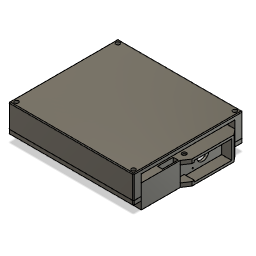
gboard_cap (Autodesk Fusion 360 design; units mm, degrees)
Autodesk Fusion 360 part; units mm, degrees
sketch "草图1" plane through (0, 0, 0) normal (0, 1, 0) x (1, 0, 0)
  line L0 (0, 0) -> (0, -50) construction
  line L1 (0, -50) -> (70, -50)
  line L2 (80, -60) -> (-80, -60)
  line L3 (-70, -50) -> (0, -50)
  line L4 (-70, 50) -> (70, 50)
  line L5 (80, 60) -> (-80, 60)
  line L6 (-70, 50) -> (-70, -50)
  line L7 (70, 50) -> (70, -50)
  line L8 (-80, 60) -> (-80, -60)
  line L9 (80, 60) -> (80, -60)
  line L10 (0, 0) -> (70, 0) construction
  line L11 (-70, 60) -> (-70, 65)
  line L12 (-70, 65) -> (-60, 65)
  line L13 (-60, 65) -> (-60, 60)
  line L14 (70, 60) -> (70, 65)
  line L15 (70, 65) -> (60, 65)
  line L16 (60, 65) -> (60, 60)
  line L17 (-70, -60) -> (-70, -65)
  line L18 (-70, -65) -> (-60, -65)
  line L19 (-60, -65) -> (-60, -60)
  line L20 (70, -60) -> (70, -65)
  line L21 (70, -65) -> (60, -65)
  line L22 (60, -65) -> (60, -60)
  dimension "d5" = 50
  dimension "d21" = 160
  dimension "d23" = 140
  dimension "d24" = 100
  dimension "d25" = 10
  dimension "d26" = 120
  dimension "d27" = 10
  dimension "d28" = 70
  dimension "d31" = 5
  dimension "d32" = 10
  dimension "d33" = 10
  dimension "d34" = 10
  dimension "d35" = 10
  dimension "d36" = 5
  dimension "d37" = 5
  dimension "d38" = 10
  dimension "d39" = 10
  dimension "d40" = 5
  dimension "d41" = 10
  dimension "d42" = 10
  constraint coincident L0.start L10.start
  constraint vertical L0
  constraint perpendicular L0 L1
  constraint perpendicular L0 L3
  constraint perpendicular L3 L6
  constraint perpendicular L1 L7
  constraint perpendicular L2 L8
  constraint perpendicular L5 L9
  constraint midpoint L7 L10.end
  constraint coincident L5 L11.start
  constraint perpendicular L5 L11
  constraint perpendicular L11 L12
  constraint coincident L5 L13.end
  constraint perpendicular L5 L13
  constraint coincident L5 L14.start
  constraint perpendicular L5 L14
  constraint perpendicular L14 L15
  constraint coincident L5 L16.end
  constraint perpendicular L5 L16
  constraint coincident L2 L17.start
  constraint perpendicular L2 L17
  constraint perpendicular L17 L18
  constraint coincident L2 L19.end
  constraint perpendicular L2 L19
  constraint coincident L2 L20.start
  constraint perpendicular L2 L20
  constraint perpendicular L20 L21
  constraint coincident L2 L22.end
  constraint perpendicular L2 L22
  measures "d5" distance of L0.start L0.end
  measures "d21" distance of L5.start L5.end
  measures "d23" distance of L6 L7
  measures "d24" distance of L3 L4
  measures "d25" distance of L7 L9
  measures "d26" distance of L2 L5
  measures "d27" distance of L4 L5
  measures "d28" distance of L0.start L10.end
  measures "d31" distance of L11.start L11.end
  measures "d32" distance of L11.end L12.end
  measures "d33" distance of L8 L11
  measures "d34" distance of L14 L16
  measures "d35" distance of L9 L14
  measures "d36" distance of L5 L15
  measures "d37" distance of L2 L21
  measures "d38" distance of L20 L22
  measures "d39" distance of L9 L20
  measures "d40" distance of L18.end L19.end
  measures "d41" distance of L17 L19
  measures "d42" distance of L8 L17
extrude "拉伸4" add sketch "草图1" along normal blind 30 makes body 1
sketch "草图6" plane through (80, 0, 0) normal (1, 0, 0) x (0, 0, -1)
  line L0 (-60, 0) -> (60, 0)
  line L1 (60, 0) -> (60, 30)
  line L2 (60, 30) -> (-60, 30)
  line L3 (-60, 30) -> (-60, 0)
  line L4 (50, 3) -> (2, 3)
  line L5 (2, 3) -> (2, 27)
  line L6 (2, 27) -> (50, 27)
  line L7 (50, 27) -> (50, 3)
  line L8 (53, 30) -> (53, 0)
  line L9 (53, 0) -> (-1, 0)
  line L10 (-1, 0) -> (-1, 30)
  line L11 (-1, 30) -> (53, 30)
  dimension "d65" = 48
  dimension "d66" = 24
  dimension "d67" = 10
  dimension "d68" = 3
  dimension "d71" = -3
  constraint horizontal L4
  constraint vertical L5
  constraint horizontal L6
  constraint vertical L7
  measures "d65" distance of L4.start L4.end
  measures "d66" distance of L4.start L6.end
  measures "d67" distance of L1 L7
  measures "d68" distance of L2 L6
extrude "拉伸9" cut sketch "草图6" against normal blind 7 contours L4 L5 L6 L7 bodies 1
extrude "拉伸10" add sketch "草图6" along normal blind 6 contours L0 L2 L8 L9 L10 L11 bodies 1
sketch "草图7" plane through (73, 0, 0) normal (1, 0, 0) x (0, 0, -1)
  line L0 (50, 27) -> (2, 27)
  line L1 (2, 27) -> (2, 3)
  line L2 (2, 3) -> (50, 3)
  line L3 (50, 3) -> (50, 27)
  line L4 (2, 15) -> (50, 15) construction
  circle A0 centre (26, 15) radius 7.5
  line L5 (50, 15) -> (13, 15) construction
  line L6 (13, 15) -> (13, 27) construction
  circle A1 centre (13, 23.5) radius 0.75
  circle A2 centre (13, 6.5) radius 0.75
  line L7 (13, 15) -> (13, 6.5) construction
  dimension "d74" = 15
  dimension "d81" = 37
  dimension "d82" = 1.5
  dimension "d83" = 3.5
  dimension "d84" = 1.5
  dimension "d85" = 3.5
  constraint midpoint L1 L4.start
  constraint midpoint L3 L4.end
  constraint midpoint L4 A0.centre
  constraint perpendicular L3 L5
  constraint coincident L0 L6.end
  constraint perpendicular L0 L6
  constraint coincident L6 A1.centre
  constraint coincident A2.centre L7.end
  constraint perpendicular L4 L7
  measures "d74" diameter of A0
  measures "d81" distance of L4.end L5.end
  measures "d82" diameter of A1
  measures "d83" distance of L0 A1.centre
  measures "d84" diameter of A2
  measures "d85" distance of L2 A2.centre
extrude "拉伸11" cut sketch "草图7" against normal blind 3 contours A0 | A1 | A2 bodies 1
sketch "草图8" plane through (0, 0, 1) normal (0, 0, 1) x (1, 0, 0)
  line L0 (80, 30) -> (80, 0)
  line L1 (80, 0) -> (86, 0)
  line L2 (86, 0) -> (86, 30)
  line L3 (86, 30) -> (80, 30)
  line L4 (86, 25) -> (80, 25)
  line L5 (80, 25) -> (80, 5)
  line L6 (80, 5) -> (86, 5)
  line L7 (86, 5) -> (86, 25)
  dimension "d77" = 5
  dimension "d78" = 5
  constraint horizontal L4
  constraint vertical L5
  constraint horizontal L6
  constraint vertical L7
  constraint coincident L0 L5.end
  constraint coincident L2 L4.start
  measures "d77" distance of L3 L4
  measures "d78" distance of L1 L6
extrude "拉伸12" cut sketch "草图8" against normal blind 3 contours L0 L2 L4 L5 L6 L7 bodies 1
sketch "草图9" plane through (0, 30, 0) normal (0, 1, 0) x (-1, 0, 0)
  line L0 (70, 50) -> (70, -50)
  line L1 (70, -50) -> (-70, -50)
  line L2 (-70, -50) -> (-70, 50)
  line L3 (-70, 50) -> (70, 50)
  line L4 (-80, -60) -> (-70, -60)
  line L5 (-70, -60) -> (-70, -65)
  line L6 (-70, -65) -> (-60, -65)
  line L7 (-60, -65) -> (-60, -60)
  line L8 (-60, -60) -> (60, -60)
  line L9 (60, -60) -> (60, -65)
  line L10 (60, -65) -> (70, -65)
  line L11 (70, -65) -> (70, -60)
  line L12 (70, -60) -> (80, -60)
  line L13 (80, -60) -> (80, 60)
  line L14 (80, 60) -> (70, 60)
  line L15 (70, 60) -> (70, 65)
  line L16 (70, 65) -> (60, 65)
  line L17 (60, 65) -> (60, 60)
  line L18 (60, 60) -> (-60, 60)
  line L19 (-60, 60) -> (-60, 65)
  line L20 (-60, 65) -> (-70, 65)
  line L21 (-70, 65) -> (-70, 60)
  line L22 (-70, 60) -> (-80, 60)
  line L23 (-80, 60) -> (-80, 1)
  line L24 (-80, 1) -> (-86, 1)
  line L25 (-86, 1) -> (-86, -53)
  line L26 (-86, -53) -> (-80, -53)
  line L27 (-80, -53) -> (-80, -60)
  line L28 (-72, 11) -> (-78.2, 11)
  line L29 (-78.2, 11) -> (-78.2, 31)
  line L30 (-78.2, 31) -> (-72, 31)
  line L31 (-72, 31) -> (-72, 11)
  line L32 (-77.2, 12) -> (-77.2, 30)
  line L33 (-77.2, 30) -> (-73, 30)
  line L34 (-73, 30) -> (-73, 12)
  line L35 (-73, 12) -> (-77.2, 12)
  dimension "d86" = 6.2
  dimension "d87" = 20
  dimension "d88" = 11
  dimension "d89" = 2
  dimension "d92" = 1
  constraint horizontal L28
  constraint vertical L29
  constraint horizontal L30
  constraint vertical L31
  measures "d86" distance of L28.start L28.end
  measures "d87" distance of L28.start L30.end
  measures "d88" distance of origin L28
  measures "d89" distance of L2 L31
extrude "拉伸13" cut sketch "草图9" against normal blind 10 contours L28 L29 L30 L31 | L32 L33 L34 L35 bodies 1
extrude "拉伸14" cut sketch "草图9" against normal blind 25 contours L32 L33 L34 L35 bodies 1
sketch "草图10" plane through (0, 0, -2) normal (0, 0, -1) x (-1, 0, 0)
  line L0 (-80, 5) -> (-86, 5)
  line L1 (-86, 5) -> (-86, 3)
  line L2 (-86, 3) -> (-73, 3)
  line L3 (-73, 3) -> (-73, 27)
  line L4 (-73, 27) -> (-86, 27)
  line L5 (-86, 27) -> (-86, 25)
  line L6 (-86, 25) -> (-80, 25)
  line L7 (-80, 25) -> (-80, 5)
  line L8 (-80, 25) -> (-73, 25)
  line L9 (-73, 25) -> (-73, 5)
  line L10 (-73, 5) -> (-80, 5)
  line L11 (-80, 5) -> (-80, 25)
  line L12 (-73, 19) -> (-78, 19)
  line L13 (-78, 19) -> (-78, 7)
  line L14 (-78, 7) -> (-73, 7)
  line L15 (-73, 7) -> (-73, 19)
  dimension "d95" = 20
  dimension "d96" = 7
  dimension "d99" = 6
  dimension "d100" = 2
  dimension "d101" = 2
  constraint horizontal L8
  constraint vertical L9
  constraint horizontal L10
  constraint vertical L11
  constraint coincident L6.end L7.start
  constraint horizontal L12
  constraint vertical L13
  constraint horizontal L14
  constraint vertical L15
  constraint coincident L9 L12.start
  measures "d95" distance of L8 L10
  measures "d96" distance of L9 L11
  measures "d99" distance of L8 L12
  measures "d100" distance of L10 L14
  measures "d101" distance of L11 L13
extrude "拉伸15" cut sketch "草图10" against normal blind 12 contours L3 L7 L8 L9 L10 L11 L12 L13 L14 | L3 L9 L12 L13 L14 L15 bodies 1
extrude "拉伸16" cut sketch "草图10" against normal up to surface (14 mm away) contours L3 L9 L12 L13 L14 L15 bodies 1
sketch "草图11" plane through (0, 0, 0) normal (0, 1, 0) x (1, 0, 0)
  line L0 (80, -1) -> (86, -1)
  line L1 (86, -1) -> (80, -10)
  line L2 (80, -10) -> (80, -1)
  line L3 (70, 50) -> (70, -50)
  line L4 (86, 53) -> (80, 53)
  line L5 (80, 60) -> (86, 53)
  line L6 (80, 53) -> (80, 60)
  dimension "d104" = 6
  dimension "d105" = 9
  dimension "d106" = 10
  dimension "d107" = 54
  dimension "d113" = 7
  constraint horizontal L0
  constraint perpendicular L0 L2
  constraint coincident L4.start L5.end
  constraint coincident L4.end L6.start
  measures "d104" distance of L0.start L0.end
  measures "d105" distance of L0.start L1.end
  measures "d106" distance of L2 L3
  measures "d107" distance of L0 L4
  measures "d113" distance of L5.start L4.end
extrude "拉伸17" add sketch "草图11" along normal blind 5 contours L0 L1 L2 bodies 1
extrude "拉伸18" add sketch "草图11" along normal blind 5 from surface at 25 contours L0 L1 L2 bodies 1
extrude "拉伸19" add sketch "草图11" along normal blind 30 contours L4 L5 L6 bodies 1
sketch "草图12" plane through (0, 30, 0) normal (0, 1, 0) x (-1, 0, 0)
  line L0 (-78.2, 11) -> (-78.2, 31)
  line L1 (-78.2, 31) -> (-72, 31)
  line L2 (-72, 31) -> (-72, 11)
  line L3 (-72, 11) -> (-78.2, 11)
  line L4 (70, 50) -> (70, -50)
  line L5 (70, -50) -> (-70, -50)
  line L6 (-70, -50) -> (-70, 50)
  line L7 (-70, 50) -> (70, 50)
  line L8 (-80, -60) -> (-70, -60)
  line L9 (-70, -60) -> (-70, -65)
  line L10 (-70, -65) -> (-60, -65)
  line L11 (-60, -65) -> (-60, -60)
  line L12 (-60, -60) -> (60, -60)
  line L13 (60, -60) -> (60, -65)
  line L14 (60, -65) -> (70, -65)
  line L15 (70, -65) -> (70, -60)
  line L16 (70, -60) -> (80, -60)
  line L17 (80, -60) -> (80, 60)
  line L18 (80, 60) -> (70, 60)
  line L19 (70, 60) -> (70, 65)
  line L20 (70, 65) -> (60, 65)
  line L21 (60, 65) -> (60, 60)
  line L22 (60, 60) -> (-60, 60)
  line L23 (-60, 60) -> (-60, 65)
  line L24 (-60, 65) -> (-70, 65)
  line L25 (-70, 65) -> (-70, 60)
  line L26 (-70, 60) -> (-80, 60)
  line L27 (-80, 60) -> (-80, 10)
  line L28 (-80, 10) -> (-86, 1)
  line L29 (-86, 1) -> (-86, -53)
  line L30 (-86, -53) -> (-80, -60)
  circle A0 centre (75, 0) radius 2.75
  circle A1 centre (-75, 0) radius 2.75
  line L31 (75, 0) -> (0, 0) construction
  dimension "d116" = 5.5
  dimension "d117" = 5.5
  dimension "d118" = 150
  dimension "d119" = 60
  dimension "d120" = 60
  dimension "d121" = 75
  constraint coincident A0.centre L31.start
  constraint coincident L31.end origin
  measures "d116" diameter of A0
  measures "d117" diameter of A1
  measures "d118" distance of A0.centre A1.centre
  measures "d119" distance of L18 A0.centre
  measures "d120" distance of L26 A1.centre
  measures "d121" distance of A0.centre L31.end
extrude "拉伸20" cut sketch "草图12" against normal blind 2 contours A0 | A1 bodies 1
sketch "草图13" plane through (0, 30, 0) normal (0, 1, 0) x (-1, 0, 0)
  circle A0 centre (75, 0) radius 2.75
  circle A1 centre (-75, 0) radius 2.75
  line L0 (-78.2, 11) -> (-78.2, 31)
  line L1 (-78.2, 31) -> (-72, 31)
  line L2 (-72, 31) -> (-72, 11)
  line L3 (-72, 11) -> (-78.2, 11)
  line L4 (70, 50) -> (70, -50)
  line L5 (70, -50) -> (-70, -50)
  line L6 (-70, -50) -> (-70, 50)
  line L7 (-70, 50) -> (70, 50)
  line L8 (-80, -60) -> (-70, -60)
  line L9 (-70, -60) -> (-70, -65)
  line L10 (-70, -65) -> (-60, -65)
  line L11 (-60, -65) -> (-60, -60)
  line L12 (-60, -60) -> (60, -60)
  line L13 (60, -60) -> (60, -65)
  line L14 (60, -65) -> (70, -65)
  line L15 (70, -65) -> (70, -60)
  line L16 (70, -60) -> (80, -60)
  line L17 (80, -60) -> (80, 60)
  line L18 (80, 60) -> (70, 60)
  line L19 (70, 60) -> (70, 65)
  line L20 (70, 65) -> (60, 65)
  line L21 (60, 65) -> (60, 60)
  line L22 (60, 60) -> (-60, 60)
  line L23 (-60, 60) -> (-60, 65)
  line L24 (-60, 65) -> (-70, 65)
  line L25 (-70, 65) -> (-70, 60)
  line L26 (-70, 60) -> (-80, 60)
  line L27 (-80, 60) -> (-80, 10)
  line L28 (-80, 10) -> (-86, 1)
  line L29 (-86, 1) -> (-86, -53)
  line L30 (-86, -53) -> (-80, -60)
  line L31 (80, -70) -> (-80, -70)
  line L32 (-80, -70) -> (-80, 70)
  line L33 (-80, 70) -> (80, 70)
  line L34 (80, 70) -> (80, -70)
  constraint perpendicular L17 L31
  constraint perpendicular L8 L32
  constraint perpendicular L32 L33
  constraint perpendicular L31 L34
extrude "拉伸21" add sketch "草图13" along normal blind 5 from surface at 10 separate body contours A0 | A1 | L0 L1 L2 L3 | L4 L5 L6 L7 | L8 L9 L10 L11 L12 L13 L14 L15 L16 L17 L18 L19 L20 L21 L22 L23 L24 L25 L26 L27 L32 L34 | L8 L9 L10 L11 L12 L13 L14 L15 L16 L31 L32 L34 | L18 L19 L20 L21 L22 L23 L24 L25 L26 L32 L33 L34 makes body 2
extrude "拉伸22" add sketch "草图13" along normal blind -15 and the other way up to surface (-10 mm away) contours L8 L9 L10 L11 L12 L13 L14 L15 L16 L31 L32 L34 | L18 L19 L20 L21 L22 L23 L24 L25 L26 L32 L33 L34 bodies 2
sketch "草图15" plane through (0, 15, 0) normal (0, -1, 0) x (1, 0, 0)
  line L0 (80, 70) -> (-80, 70)
  line L1 (-80, 70) -> (-80, 60)
  line L2 (-80, 60) -> (-70, 60)
  line L3 (-70, 60) -> (-70, 65)
  line L4 (-70, 65) -> (-60, 65)
  line L5 (-60, 65) -> (-60, 60)
  line L6 (-60, 60) -> (60, 60)
  line L7 (60, 60) -> (60, 65)
  line L8 (60, 65) -> (70, 65)
  line L9 (70, 65) -> (70, 60)
  line L10 (70, 60) -> (80, 60)
  line L11 (80, 60) -> (80, 70)
  line L12 (-80, 70) -> (80, 70)
  line L13 (80, 70) -> (80, 60)
  line L14 (80, 60) -> (-80, 60)
  line L15 (-80, 60) -> (-80, 70)
  line L16 (-80, -60) -> (80, -60)
  line L17 (80, -60) -> (80, -70)
  line L18 (80, -70) -> (-80, -70)
  line L19 (-80, -70) -> (-80, -60)
  constraint horizontal L12
  constraint vertical L13
  constraint horizontal L14
  constraint vertical L15
  constraint coincident L10.end L11.start
  constraint coincident L0.end L1.start
  constraint horizontal L16
  constraint vertical L17
  constraint horizontal L18
  constraint vertical L19
extrude "拉伸24" add sketch "草图15" along normal blind 5 separate body makes body 3 at (-26.6667, 15, -63.3333) makes body 4 at (26.6667, 15, 63.3333)
sketch "草图16" plane through (0, 10, 0) normal (0, -1, 0) x (1, 0, 0)
  line L0 (-80, 60) -> (80, 60)
  line L1 (80, 60) -> (80, 70)
  line L2 (80, 70) -> (-80, 70)
  line L3 (-80, 70) -> (-80, 60)
  circle A0 centre (-75, 65) radius 3.25
  circle A1 centre (-75, 65) radius 1.35
  line L4 (-75, 65) -> (-75, 0) construction
  line L5 (-75, 0) -> (0, 0) construction
  circle A2 centre (75, 65) radius 3.25
  circle A3 centre (75, 65) radius 1.35
  circle A4 centre (-75, -65) radius 3.25
  circle A5 centre (-75, -65) radius 1.35
  circle A6 centre (75, -65) radius 3.25
  circle A7 centre (75, -65) radius 1.35
  dimension "d135" = 6.5
  dimension "d136" = 2.7
  dimension "d137" = 65
  dimension "d138" = 75
  dimension "d141" = 150
  dimension "d142" = -130
  constraint concentric A0 A1
  constraint coincident A0.centre A1.centre
  constraint parallel L3 L4
  constraint coincident L5.end origin
  constraint perpendicular L4 L5
  measures "d135" diameter of A0
  measures "d136" diameter of A1
  measures "d137" distance of A0.centre L4.end
  measures "d138" distance of L4.end L5.end
extrude "拉伸25" cut sketch "草图16" against normal blind 2 contours A0 | A1 | A2 | A3 | A4 | A5 | A6 | A7 bodies 1 4
extrude "拉伸26" cut sketch "草图16" against normal blind 9 contours A1 | A3 | A5 | A7 bodies 2 3 4
sketch "草图17" plane through (0, 45, 0) normal (0, 1, 0) x (-1, 0, 0)
  line L0 (80, 70) -> (-80, 70)
  line L1 (-80, 70) -> (-80, -70)
  line L2 (-80, -70) -> (80, -70)
  line L3 (80, -70) -> (80, 70)
  circle A0 centre (75, 65) radius 2.5
  line L4 (0, 0) -> (75, 0) construction
  line L5 (75, 0) -> (75, 65) construction
  circle A1 centre (-75, 65) radius 2.5
  circle A2 centre (75, -65) radius 2.5
  circle A3 centre (-75, -65) radius 2.5
  dimension "d150" = 5
  dimension "d151" = 75
  dimension "d152" = 65
  dimension "d155" = -150
  dimension "d156" = -130
  constraint coincident L4.start origin
  constraint horizontal L4
  constraint coincident A0.centre L5.end
  constraint perpendicular L4 L5
  measures "d150" diameter of A0
  measures "d151" distance of L4.start L4.end
  measures "d152" distance of L4.end A0.centre
extrude "拉伸27" cut sketch "草图17" against normal blind 5 contours A0 | A1 | A2 | A3 bodies 2
fillet "圆角1" radius 1 12 edges at (0, 45, 70) (-80, 45, 0) (-80, 30, 70) (80, 30, 70) (80, 45, 0) (0, 45, -70) (80, 30, -70) (-80, 30, -70) (80, 12.5, -70) (-80, 12.5, -70) (-80, 12.5, 70) (80, 12.5, 70) on bodies 2 3 4
sketch "草图18" plane through (0, 0, 65) normal (0, 0, 1) x (1, 0, 0)
  line L0 (-70, 0) -> (-60, 0)
  line L1 (-60, 0) -> (-60, 30)
  line L2 (-60, 30) -> (-70, 30)
  line L3 (-70, 30) -> (-70, 0)
  line L4 (-70, 15) -> (-60, 15)
  line L5 (-60, 15) -> (-60, 0)
  line L6 (-60, 0) -> (-70, 0)
  line L7 (-70, 0) -> (-70, 15)
  line L8 (70, 0) -> (60, 0)
  line L9 (60, 0) -> (60, 15)
  line L10 (60, 15) -> (70, 15)
  line L11 (70, 15) -> (70, 0)
  dimension "d161" = 120
  dimension "d162" = 15
  dimension "d163" = 10
  dimension "d164" = 15
  constraint horizontal L4
  constraint vertical L5
  constraint horizontal L6
  constraint vertical L7
  constraint coincident L0.end L1.start
  constraint midpoint L3 L4.start
  constraint horizontal L8
  constraint vertical L9
  constraint horizontal L10
  constraint vertical L11
  measures "d161" distance of L5 L9
  measures "d162" distance of L8 L10
  measures "d163" distance of L9 L11
  measures "d164" distance of origin L10
extrude "拉伸28" cut sketch "草图18" against normal blind 5 contours L0 L1 L3 L4 L5 L6 L7 | L8 L9 L10 L11 bodies 1
extrude "拉伸29" cut sketch "草图18" against normal blind 5 from surface at -125 contours L0 L1 L3 L4 L5 L6 L7 | L8 L9 L10 L11 bodies 1
extrude "拉伸30" cut sketch "草图12" along normal blind 12 contours A0 | A1 bodies 2
sketch "草图19" plane through (0, 0, 0) normal (0, 0, 1) x (1, 0, 0)
